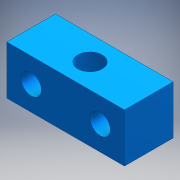
# Autodesk Inventor part: smallSprocketFixture
Saved by Autodesk Inventor 2016 (Build 200138000, 138)
## iProperties
Created: 2016-05-21
Part Number: smallSprocketFixture
Material: ABS Plastic
Document SubType Name: Modeling
Designer: Henrik Samuelsson
Density: 1.06 g/cm^3
Appearance: Smooth - White
Author: Henrik Samuelsson
Autodesk Inventor part; units mm, degrees
ref_plane "YZ Plane" through (0, 0, 0) normal (1, 0, 0) x (0, 1, 0)
ref_plane "XZ Plane" through (0, 0, 0) normal (0, 1, 0) x (-1, 0, 0)
ref_plane "XY Plane" through (0, 0, 0) normal (0, 0, 1) x (1, 0, 0)
sketch "Sketch1" plane through (0, 0, 0) normal (0, 1, 0) x (-1, 0, 0)
  line L0 (0, 0) -> (29, 0)
  line L1 (29, 0) -> (29, -12)
  line L2 (29, -12) -> (0, -12)
  line L3 (0, -12) -> (0, 0)
  circle A0 centre (23, -6) radius 2.5
  circle A1 centre (6, -6) radius 2.5
  dimension "d0" = 12
  dimension "d1" = 29
  dimension "d2" = 5
  dimension "d3" = 5
  dimension "d4" = 6
  dimension "d6" = 6
  dimension "d7" = 6
  dimension "d9" = 17
  constraints: 8 end point, 2 centre point, 2 parallel, 1 horizontal, 1 perpendicular
  measures "d0" distance of L1.end L0.end
  measures "d1" distance of L2.end L1.end
  measures "d2" diameter of A0
  measures "d3" diameter of A1
  measures "d4" distance from line of L1 A0.centre
  measures "d6" distance from line of L2 A1.centre
  measures "d7" distance from line of L2 A0.centre
  measures "d9" distance of A0.centre A1.centre
extrude "Extrusion1" add sketch "Sketch1" along normal blind 12
sketch "Sketch2" plane through (0, 0, -12) normal (0, 0, -1) x (-1, 0, 0)
  circle A0 centre (14.5, 6) radius 3
  line L0 (29, 0) -> (29, 12) projected
  point P0 (0, 0)
  dimension "d12" = 6
  dimension "d13" = 6
  dimension "d14" = 14.5
  constraints: 1 centre point
  measures "d12" diameter of A0
  measures "d13" vertical distance of point (0, 0) A0.centre
  measures "d14" distance from line of L0 A0.centre
extrude "Extrusion2" cut sketch "Sketch2" against normal up to next
body "Solid1"
